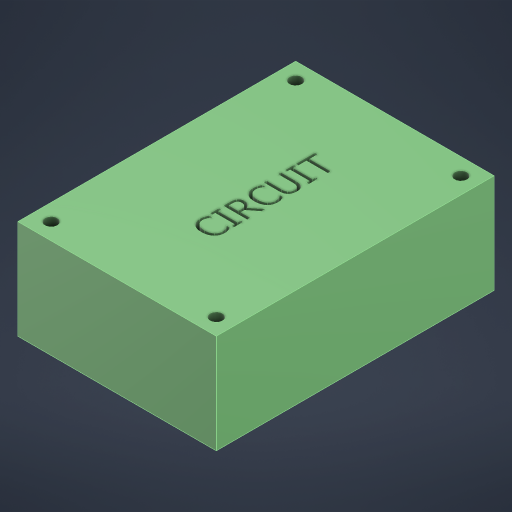
# Autodesk Inventor part: Circuit
Saved by Autodesk Inventor 2024.3 (Build 283343000, 343)
## iProperties
Created: 2022-08-23
Part Number: Circuit
Material: PMMA 플라스틱
Document SubType Name: Modeling
Designer: awind
Density: 1.188 g/cm^3
Appearance: 매끄러움 - 짙은 산림 녹색
Mass: 101.085 g
Surface Area: 182.531 cm^2
Volume: 85.0882 cm^3
Author: awind
Autodesk Inventor part; units mm, degrees
ref_plane "YZ Plane" through (0, 0, 0) normal (1, 0, 0) x (0, 1, 0)
ref_plane "XZ Plane" through (0, 0, 0) normal (0, 1, 0) x (-1, 0, 0)
ref_plane "XY Plane" through (0, 0, 0) normal (0, 0, 1) x (1, 0, 0)
sketch "스케치1" plane through (0, 0, 0) normal (0, 1, 0) x (-1, 0, 0)
  line L0 (25, 35) -> (-25, 35)
  line L1 (-25, 35) -> (-25, -35)
  line L2 (-25, -35) -> (25, -35)
  line L3 (25, -35) -> (25, 35)
  line L4 (25, 35) -> (-25, -35) construction
  line L5 (-25, 35) -> (25, -35) construction
  point P0 (0, 0)
  dimension "d0" = 50
  dimension "d1" = 70
  constraints: 12 end point, 2 midpoint, 2 parallel, 1 horizontal, 1 perpendicular
  measures "d0" distance of L2.end L1.end
  measures "d1" distance of L1.end L0.end
extrude "돌출1" add sketch "스케치1" along normal blind 25
sketch "스케치3" plane through (0, 25, 0) normal (0, 1, 0) x (1, 0, 0)
  line L0 (-2.7479, -14.4503) -> (-2.7479, 8.7197) construction
  line L1 (-2.7479, 8.7197) -> (8.9074, 8.7197) construction
  line L2 (8.9074, 8.7197) -> (8.9074, -14.4503) construction
  line L3 (8.9074, -14.4503) -> (-2.7479, -14.4503) construction
  spline S0 degree 2 poles (3.5696, -11.4498) (3.5696, -12.043) (3.1692, -13.0464) (2.7688, -13.4123) knots 0 0 0 1 2 2 2
  spline S1 degree 2 poles (2.7688, -13.4123) (2.3733, -13.7781) (1.187, -14.1785) (0.4158, -14.1785) knots 0 0 0 1 2 2 2
  spline S2 degree 2 poles (0.4158, -14.1785) (-0.3504, -14.1785) (-1.4874, -13.7879) (-1.9075, -13.4172) knots 0 0 0 1 2 2 2
  spline S3 degree 2 poles (-1.9075, -13.4172) (-2.3178, -13.0514) (-2.7479, -12.0529) (-2.7479, -11.4349) knots 0 0 0 1 2 2 2
  spline S4 degree 2 poles (-2.7479, -11.4349) (-2.7479, -11.1285) (-2.6589, -10.5896) (-2.5897, -10.3623) knots 0 0 0 1 2 2 2
  spline S5 degree 2 poles (-2.5897, -10.3623) (-2.5254, -10.1645) (-2.3425, -9.7542) (-2.2338, -9.5516) knots 0 0 0 1 2 2 2
  line L4 (-2.2338, -9.5516) -> (-1.255, -9.5516)
  line L5 (-1.255, -9.5516) -> (-1.255, -9.6158)
  spline S6 degree 2 poles (-1.255, -9.6158) (-1.3539, -9.7246) (-1.6307, -10.0607) (-1.7642, -10.3029) knots 0 0 0 1 2 2 2
  spline S7 degree 2 poles (-1.7642, -10.3029) (-1.8927, -10.5353) (-2.0558, -11.084) (-2.0558, -11.4399) knots 0 0 0 1 2 2 2
  spline S8 degree 2 poles (-2.0558, -11.4399) (-2.0558, -11.8304) (-1.7345, -12.5274) (-1.428, -12.7894) knots 0 0 0 1 2 2 2
  spline S9 degree 2 poles (-1.428, -12.7894) (-1.1166, -13.0464) (-0.1724, -13.3332) (0.4158, -13.3332) knots 0 0 0 1 2 2 2
  spline S10 degree 2 poles (0.4158, -13.3332) (1.0436, -13.3332) (1.9482, -13.0316) (2.2596, -12.7696) knots 0 0 0 1 2 2 2
  spline S11 degree 2 poles (2.2596, -12.7696) (2.5612, -12.5126) (2.8677, -11.8255) (2.8677, -11.4399) knots 0 0 0 1 2 2 2
  spline S12 degree 2 poles (2.8677, -11.4399) (2.8677, -11.0889) (2.6947, -10.4908) (2.5661, -10.2584) knots 0 0 0 1 2 2 2
  spline S13 degree 2 poles (2.5661, -10.2584) (2.4376, -10.036) (2.1707, -9.7048) (2.0767, -9.6109) knots 0 0 0 1 2 2 2
  line L6 (2.0767, -9.6109) -> (2.0767, -9.5516)
  line L7 (2.0767, -9.5516) -> (3.0456, -9.5516)
  spline S14 degree 2 poles (3.0456, -9.5516) (3.1396, -9.7542) (3.3126, -10.1101) (3.3917, -10.3623) knots 0 0 0 1 2 2 2
  spline S15 degree 2 poles (3.3917, -10.3623) (3.4806, -10.6292) (3.5696, -11.084) (3.5696, -11.4498) knots 0 0 0 1 2 2 2
  line L8 (3.4609, -6.6696) -> (3.4609, -9.0325)
  line L9 (3.4609, -9.0325) -> (2.838, -9.0325)
  line L10 (2.838, -9.0325) -> (2.838, -8.2564)
  line L11 (2.838, -8.2564) -> (-2.0163, -8.2564)
  line L12 (-2.0163, -8.2564) -> (-2.0163, -9.0325)
  line L13 (-2.0163, -9.0325) -> (-2.6391, -9.0325)
  line L14 (-2.6391, -9.0325) -> (-2.6391, -6.6696)
  line L15 (-2.6391, -6.6696) -> (-2.0163, -6.6696)
  line L16 (-2.0163, -6.6696) -> (-2.0163, -7.4457)
  line L17 (-2.0163, -7.4457) -> (2.838, -7.4457)
  line L18 (2.838, -7.4457) -> (2.838, -6.6696)
  line L19 (2.838, -6.6696) -> (3.4609, -6.6696)
  line L20 (3.4609, -0.9453) -> (3.4609, -1.9982)
  line L21 (3.4609, -1.9982) -> (1.0337, -3.9261)
  line L22 (1.0337, -3.9261) -> (1.0337, -4.8554)
  line L23 (1.0337, -4.8554) -> (3.4609, -4.8554)
  line L24 (3.4609, -4.8554) -> (3.4609, -5.6661)
  line L25 (3.4609, -5.6661) -> (-2.6391, -5.6661)
  line L26 (-2.6391, -5.6661) -> (-2.6391, -4.0942)
  spline S16 degree 2 poles (-2.6391, -4.0942) (-2.6391, -3.5702) (-2.5254, -2.8633) (-2.3178, -2.542) knots 0 0 0 1 2 2 2
  spline S17 degree 2 poles (-2.3178, -2.542) (-2.1102, -2.2207) (-1.4626, -1.8499) (-0.9831, -1.8499) knots 0 0 0 1 2 2 2
  spline S18 degree 2 poles (-0.9831, -1.8499) (-0.3158, -1.8499) (0.5888, -2.5321) (0.8063, -3.1154) knots 0 0 0 1 2 2 2
  line L27 (0.8063, -3.1154) -> (3.4609, -0.9453)
  spline S19 degree 2 poles (-0.9189, -2.6952) (-1.1858, -2.6952) (-1.5961, -2.8831) (-1.7296, -3.0808) knots 0 0 0 1 2 2 2
  spline S20 degree 2 poles (-1.7296, -3.0808) (-1.8433, -3.2538) (-1.9372, -3.7135) (-1.9372, -4.0497) knots 0 0 0 1 2 2 2
  line L28 (-1.9372, -4.0497) -> (-1.9372, -4.8554)
  line L29 (-1.9372, -4.8554) -> (0.3565, -4.8554)
  line L30 (0.3565, -4.8554) -> (0.3565, -4.1436)
  spline S21 degree 2 poles (0.3565, -4.1436) (0.3565, -3.7926) (0.2329, -3.2341) (0.0401, -3.0413) knots 0 0 0 1 2 2 2
  spline S22 degree 2 poles (0.0401, -3.0413) (-0.128, -2.8633) (-0.6025, -2.6952) (-0.9189, -2.6952) knots 0 0 0 1 2 2 2
  spline S23 degree 2 poles (3.5696, 1.9218) (3.5696, 1.3286) (3.1692, 0.3251) (2.7688, -0.0407) knots 0 0 0 1 2 2 2
  spline S24 degree 2 poles (2.7688, -0.0407) (2.3733, -0.4065) (1.187, -0.8069) (0.4158, -0.8069) knots 0 0 0 1 2 2 2
  spline S25 degree 2 poles (0.4158, -0.8069) (-0.3504, -0.8069) (-1.4874, -0.4164) (-1.9075, -0.0456) knots 0 0 0 1 2 2 2
  spline S26 degree 2 poles (-1.9075, -0.0456) (-2.3178, 0.3202) (-2.7479, 1.3187) (-2.7479, 1.9366) knots 0 0 0 1 2 2 2
  spline S27 degree 2 poles (-2.7479, 1.9366) (-2.7479, 2.2431) (-2.6589, 2.7819) (-2.5897, 3.0093) knots 0 0 0 1 2 2 2
  spline S28 degree 2 poles (-2.5897, 3.0093) (-2.5254, 3.207) (-2.3425, 3.6173) (-2.2338, 3.82) knots 0 0 0 1 2 2 2
  line L31 (-2.2338, 3.82) -> (-1.255, 3.82)
  line L32 (-1.255, 3.82) -> (-1.255, 3.7557)
  spline S29 degree 2 poles (-1.255, 3.7557) (-1.3539, 3.647) (-1.6307, 3.3108) (-1.7642, 3.0686) knots 0 0 0 1 2 2 2
  spline S30 degree 2 poles (-1.7642, 3.0686) (-1.8927, 2.8363) (-2.0558, 2.2876) (-2.0558, 1.9317) knots 0 0 0 1 2 2 2
  spline S31 degree 2 poles (-2.0558, 1.9317) (-2.0558, 1.5412) (-1.7345, 0.8442) (-1.428, 0.5822) knots 0 0 0 1 2 2 2
  spline S32 degree 2 poles (-1.428, 0.5822) (-1.1166, 0.3251) (-0.1724, 0.0384) (0.4158, 0.0384) knots 0 0 0 1 2 2 2
  spline S33 degree 2 poles (0.4158, 0.0384) (1.0436, 0.0384) (1.9482, 0.3399) (2.2596, 0.6019) knots 0 0 0 1 2 2 2
  spline S34 degree 2 poles (2.2596, 0.6019) (2.5612, 0.859) (2.8677, 1.5461) (2.8677, 1.9317) knots 0 0 0 1 2 2 2
  spline S35 degree 2 poles (2.8677, 1.9317) (2.8677, 2.2826) (2.6947, 2.8808) (2.5661, 3.1131) knots 0 0 0 1 2 2 2
  spline S36 degree 2 poles (2.5661, 3.1131) (2.4376, 3.3356) (2.1707, 3.6668) (2.0767, 3.7607) knots 0 0 0 1 2 2 2
  line L33 (2.0767, 3.7607) -> (2.0767, 3.82)
  line L34 (2.0767, 3.82) -> (3.0456, 3.82)
  spline S37 degree 2 poles (3.0456, 3.82) (3.1396, 3.6173) (3.3126, 3.2614) (3.3917, 3.0093) knots 0 0 0 1 2 2 2
  spline S38 degree 2 poles (3.3917, 3.0093) (3.4806, 2.7424) (3.5696, 2.2876) (3.5696, 1.9218) knots 0 0 0 1 2 2 2
  spline S39 degree 2 poles (3.5894, 6.7069) (3.5894, 6.1681) (3.3076, 5.3672) (3.0259, 5.0855) knots 0 0 0 1 2 2 2
  spline S40 degree 2 poles (3.0259, 5.0855) (2.7095, 4.7642) (1.8197, 4.5022) (1.1672, 4.5022) knots 0 0 0 1 2 2 2
  line L35 (1.1672, 4.5022) -> (-2.6391, 4.5022)
  line L36 (-2.6391, 4.5022) -> (-2.6391, 5.3129)
  line L37 (-2.6391, 5.3129) -> (1.1672, 5.3129)
  spline S41 degree 2 poles (1.1672, 5.3129) (1.5923, 5.3129) (2.1657, 5.4216) (2.3981, 5.5749) knots 0 0 0 1 2 2 2
  spline S42 degree 2 poles (2.3981, 5.5749) (2.6452, 5.738) (2.8973, 6.3015) (2.8973, 6.7069) knots 0 0 0 1 2 2 2
  spline S43 degree 2 poles (2.8973, 6.7069) (2.8973, 7.0875) (2.6452, 7.6807) (2.3981, 7.8438) knots 0 0 0 1 2 2 2
  spline S44 degree 2 poles (2.3981, 7.8438) (2.1657, 7.9971) (1.5972, 8.1058) (1.187, 8.1058) knots 0 0 0 1 2 2 2
  line L38 (1.187, 8.1058) -> (-2.6391, 8.1058)
  line L39 (-2.6391, 8.1058) -> (-2.6391, 8.9165)
  line L40 (-2.6391, 8.9165) -> (1.1672, 8.9165)
  spline S45 degree 2 poles (1.1672, 8.9165) (1.8049, 8.9165) (2.7144, 8.6595) (3.0259, 8.3332) knots 0 0 0 1 2 2 2
  spline S46 degree 2 poles (3.0259, 8.3332) (3.3126, 8.0416) (3.5894, 7.2704) (3.5894, 6.7069) knots 0 0 0 1 2 2 2
  line L41 (3.4609, 12.2038) -> (3.4609, 9.8409)
  line L42 (3.4609, 9.8409) -> (2.838, 9.8409)
  line L43 (2.838, 9.8409) -> (2.838, 10.617)
  line L44 (2.838, 10.617) -> (-2.0163, 10.617)
  line L45 (-2.0163, 10.617) -> (-2.0163, 9.8409)
  line L46 (-2.0163, 9.8409) -> (-2.6391, 9.8409)
  line L47 (-2.6391, 9.8409) -> (-2.6391, 12.2038)
  line L48 (-2.6391, 12.2038) -> (-2.0163, 12.2038)
  line L49 (-2.0163, 12.2038) -> (-2.0163, 11.4277)
  line L50 (-2.0163, 11.4277) -> (2.838, 11.4277)
  line L51 (2.838, 11.4277) -> (2.838, 12.2038)
  line L52 (2.838, 12.2038) -> (3.4609, 12.2038)
  line L53 (3.4609, 14.6309) -> (-1.9174, 14.6309)
  line L54 (-1.9174, 14.6309) -> (-1.9174, 12.5844)
  line L55 (-1.9174, 12.5844) -> (-2.6391, 12.5844)
  line L56 (-2.6391, 12.5844) -> (-2.6391, 17.4882)
  line L57 (-2.6391, 17.4882) -> (-1.9174, 17.4882)
  line L58 (-1.9174, 17.4882) -> (-1.9174, 15.4416)
  line L59 (-1.9174, 15.4416) -> (3.4609, 15.4416)
  line L60 (3.4609, 15.4416) -> (3.4609, 14.6309)
  point P0 (0, 0)
  constraints: 2 other
extrude "돌출3" cut sketch "스케치3" against normal blind 30
sketch "스케치4" plane through (0, 25, 0) normal (0, 1, 0) x (1, 0, 0)
  line L0 (25, -35) -> (25, 35) projected
  line L1 (25, 35) -> (-25, 35) projected
  line L2 (-25, 35) -> (-25, -35) projected
  line L3 (-25, -35) -> (25, -35) projected
  line L4 (3.4609, 15.4416) -> (3.4609, 14.6309) projected
  line L5 (3.4609, 14.6309) -> (-1.9174, 14.6309) projected
  line L6 (-1.9174, 14.6309) -> (-1.9174, 12.5844) projected
  line L7 (-1.9174, 12.5844) -> (-2.6391, 12.5844) projected
  line L8 (-2.6391, 12.5844) -> (-2.6391, 17.4882) projected
  line L9 (-2.6391, 17.4882) -> (-1.9174, 17.4882) projected
  line L10 (-1.9174, 17.4882) -> (-1.9174, 15.4416) projected
  line L11 (-1.9174, 15.4416) -> (3.4609, 15.4416) projected
  line L12 (1.1672, 4.5022) -> (-2.6391, 4.5022) projected
  line L13 (-2.6391, 4.5022) -> (-2.6391, 5.3129) projected
  line L14 (-2.6391, 5.3129) -> (1.1672, 5.3129) projected
  line L15 (1.187, 8.1058) -> (-2.6391, 8.1058) projected
  line L16 (-2.6391, 8.1058) -> (-2.6391, 8.9165) projected
  line L17 (-2.6391, 8.9165) -> (1.1672, 8.9165) projected
  line L18 (2.838, -6.6696) -> (3.4609, -6.6696) projected
  line L19 (3.4609, -6.6696) -> (3.4609, -9.0325) projected
  line L20 (3.4609, -9.0325) -> (2.838, -9.0325) projected
  line L21 (2.838, -9.0325) -> (2.838, -8.2564) projected
  line L22 (2.838, -8.2564) -> (-2.0163, -8.2564) projected
  line L23 (-2.0163, -8.2564) -> (-2.0163, -9.0325) projected
  line L24 (-2.0163, -9.0325) -> (-2.6391, -9.0325) projected
  line L25 (-2.6391, -9.0325) -> (-2.6391, -6.6696) projected
  line L26 (-2.6391, -6.6696) -> (-2.0163, -6.6696) projected
  line L27 (-2.0163, -6.6696) -> (-2.0163, -7.4457) projected
  line L28 (-2.0163, -7.4457) -> (2.838, -7.4457) projected
  line L29 (2.838, -7.4457) -> (2.838, -6.6696) projected
  line L30 (-2.2338, -9.5516) -> (-1.255, -9.5516) projected
  line L31 (-1.255, -9.5516) -> (-1.255, -9.6158) projected
  line L32 (2.0767, -9.6109) -> (2.0767, -9.5516) projected
  line L33 (2.0767, -9.5516) -> (3.0456, -9.5516) projected
  line L34 (0.8063, -3.1154) -> (3.4609, -0.9453) projected
  line L35 (3.4609, -0.9453) -> (3.4609, -1.9982) projected
  line L36 (3.4609, -1.9982) -> (1.0337, -3.9261) projected
  line L37 (1.0337, -3.9261) -> (1.0337, -4.8554) projected
  line L38 (1.0337, -4.8554) -> (3.4609, -4.8554) projected
  line L39 (3.4609, -4.8554) -> (3.4609, -5.6661) projected
  line L40 (3.4609, -5.6661) -> (-2.6391, -5.6661) projected
  line L41 (-2.6391, -5.6661) -> (-2.6391, -4.0942) projected
  line L42 (-2.2338, 3.82) -> (-1.255, 3.82) projected
  line L43 (-1.255, 3.82) -> (-1.255, 3.7557) projected
  line L44 (2.0767, 3.7607) -> (2.0767, 3.82) projected
  line L45 (2.0767, 3.82) -> (3.0456, 3.82) projected
  line L46 (2.838, 12.2038) -> (3.4609, 12.2038) projected
  line L47 (3.4609, 12.2038) -> (3.4609, 9.8409) projected
  line L48 (3.4609, 9.8409) -> (2.838, 9.8409) projected
  line L49 (2.838, 9.8409) -> (2.838, 10.617) projected
  line L50 (2.838, 10.617) -> (-2.0163, 10.617) projected
  line L51 (-2.0163, 10.617) -> (-2.0163, 9.8409) projected
  line L52 (-2.0163, 9.8409) -> (-2.6391, 9.8409) projected
  line L53 (-2.6391, 9.8409) -> (-2.6391, 12.2038) projected
  line L54 (-2.6391, 12.2038) -> (-2.0163, 12.2038) projected
  line L55 (-2.0163, 12.2038) -> (-2.0163, 11.4277) projected
  line L56 (-2.0163, 11.4277) -> (2.838, 11.4277) projected
  line L57 (2.838, 11.4277) -> (2.838, 12.2038) projected
  circle A0 centre (-20.8, -30.8) radius 1.6
  circle A1 centre (20.8, -30.8) radius 1.6
  circle A2 centre (-20.8, 30.8) radius 1.6
  circle A3 centre (20.8, 30.8) radius 1.6
  point P0 (0, 0)
  point P1 (3.0259, 8.3332)
  point P2 (3.5894, 6.7069)
  point P3 (3.0259, 5.0855)
  point P4 (2.3981, 5.5749)
  point P5 (2.8973, 6.7069)
  point P6 (2.3981, 7.8438)
  point P7 (3.3917, -10.3623)
  point P8 (3.5696, -11.4498)
  point P9 (2.7688, -13.4123)
  point P10 (0.4158, -14.1785)
  point P11 (-1.9075, -13.4172)
  point P12 (-2.7479, -11.4349)
  point P13 (-2.5897, -10.3623)
  point P14 (-1.7642, -10.3029)
  point P15 (-2.0558, -11.4399)
  point P16 (-1.428, -12.7894)
  point P17 (0.4158, -13.3332)
  point P18 (2.2596, -12.7696)
  point P19 (2.8677, -11.4399)
  point P20 (2.5661, -10.2584)
  point P21 (-2.3178, -2.542)
  point P22 (-0.9831, -1.8499)
  point P23 (3.3917, 3.0093)
  point P24 (3.5696, 1.9218)
  point P25 (2.7688, -0.0407)
  point P26 (0.4158, -0.8069)
  point P27 (-1.9075, -0.0456)
  point P28 (-2.7479, 1.9366)
  point P29 (-2.5897, 3.0093)
  point P30 (-1.7642, 3.0686)
  point P31 (-2.0558, 1.9317)
  point P32 (-1.428, 0.5822)
  point P33 (0.4158, 0.0384)
  point P34 (2.2596, 0.6019)
  point P35 (2.8677, 1.9317)
  point P36 (2.5661, 3.1131)
  dimension "d19" = 3.2
  dimension "d20" = 4.2
  dimension "d21" = 4.2
  dimension "d22" = 3.2
  dimension "d23" = 4.2
  dimension "d24" = 4.2
  dimension "d25" = 3.2
  dimension "d26" = 3.2
  dimension "d27" = 4.2
  dimension "d28" = 4.2
  dimension "d29" = 4.2
  dimension "d30" = 4.2
  constraints: 4 centre point, 43 other
  measures "d19" diameter of A0
  measures "d20" distance from line of L2 A0.centre
  measures "d21" distance from line of L3 A0.centre
  measures "d22" diameter of A1
  measures "d23" distance from line of L3 A1.centre
  measures "d24" distance from line of L0 A1.centre
  measures "d25" diameter of A2
  measures "d26" diameter of A3
  measures "d27" distance from line of L1 A3.centre
  measures "d28" distance from line of L0 A3.centre
  measures "d29" distance from line of L2 A2.centre
  measures "d30" distance from line of L1 A2.centre
extrude "돌출4" cut sketch "스케치4" against normal through all contours A0 | A1 | A2 | A3
